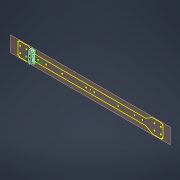
# Autodesk Inventor part: Home Switch Mount X
Saved by Autodesk Inventor 2022 (Build 260153000, 153)
## iProperties
Created: 2021-11-21
Part Number: Home Switch Mount X
Material: Generic
Document SubType Name: Modeling
Designer: nicol
Density: 1 g/cm^3
Appearance: Default
Author: nicol
Autodesk Inventor part; units mm, degrees
ref_plane "YZ Plane" through (0, 0, 0) normal (1, 0, 0) x (0, 1, 0)
ref_plane "XZ Plane" through (0, 0, 0) normal (0, 1, 0) x (-1, 0, 0)
ref_plane "XY Plane" through (0, 0, 0) normal (0, 0, 1) x (1, 0, 0)
ref_plane "Work Plane1" through (0, 0, 0) normal (0, 0, 1) x (1, 0, 0)
sketch "Sketch1" plane through (0, 0, 0) normal (0, 0, 1) x (1, 0, 0)
  line L0 (-193.5, -22) -> (-172.7154, -10) projected
  arc A0 (-226.5, -17.6844) -> (-226.2768, -18.2232) centre (-225.738, -17.6844) ccw projected
  line L1 (-222.7232, -21.7768) -> (-226.2768, -18.2232) projected
  arc A1 (-222.7232, -21.7768) -> (-222.1844, -22) centre (-222.1844, -21.238) ccw projected
  line L2 (-193.5, -22) -> (-222.1844, -22) projected
  line L3 (-193.5, -22) -> (-172.7154, -10) projected
  line L4 (-172.7154, -10) -> (172.7154, -10) projected
  line L5 (172.7154, -10) -> (193.5, -22) projected
  line L6 (193.5, -22) -> (222.1844, -22) projected
  arc A2 (222.1844, -22) -> (222.7232, -21.7768) centre (222.1844, -21.238) ccw projected
  line L7 (226.2768, -18.2232) -> (222.7232, -21.7768) projected
  arc A3 (226.2768, -18.2232) -> (226.5, -17.6844) centre (225.738, -17.6844) ccw projected
  line L8 (226.5, 17.6844) -> (226.5, -17.6844) projected
  arc A4 (226.5, 17.6844) -> (226.2768, 18.2232) centre (225.738, 17.6844) ccw projected
  line L9 (222.7232, 21.7768) -> (226.2768, 18.2232) projected
  arc A5 (222.7232, 21.7768) -> (222.1844, 22) centre (222.1844, 21.238) ccw projected
  line L10 (193.5, 22) -> (222.1844, 22) projected
  line L11 (193.5, 22) -> (172.7154, 10) projected
  line L12 (172.7154, 10) -> (-172.7154, 10) projected
  line L13 (-172.7154, 10) -> (-193.5, 22) projected
  line L14 (-193.5, 22) -> (-222.1844, 22) projected
  arc A6 (-222.1844, 22) -> (-222.7232, 21.7768) centre (-222.1844, 21.238) ccw projected
  line L15 (-226.2768, 18.2232) -> (-222.7232, 21.7768) projected
  arc A7 (-226.2768, 18.2232) -> (-226.5, 17.6844) centre (-225.738, 17.6844) ccw projected
  line L16 (-226.5, -17.6844) -> (-226.5, 17.6844) projected
  circle A8 centre (-13, 0) radius 1.2645 projected
  circle A9 centre (87, 0) radius 1.2645 projected
  circle A10 centre (-138, 0) radius 1.2645 projected
  circle A11 centre (162, 0) radius 1.2645 projected
  circle A12 centre (-163, 0) radius 1.2645 projected
  circle A13 centre (137, 0) radius 1.2645 projected
  circle A14 centre (-88, 0) radius 1.2645 projected
  circle A15 centre (12, 0) radius 1.2645 projected
  circle A16 centre (-200, -10) radius 1.7 projected
  circle A17 centre (-220, 10) radius 1.7 projected
  circle A18 centre (-220, -10) radius 1.7 projected
  circle A19 centre (-200, 10) radius 1.7 projected
  circle A20 centre (200, -10) radius 1.7 projected
  circle A21 centre (220, 10) radius 1.7 projected
  circle A22 centre (220, -10) radius 1.7 projected
  circle A23 centre (200, 10) radius 1.7 projected
  line L17 (-175, -5.5) -> (-175, 5.5) projected
  line L18 (-187.7, -18.6514) -> (-175, -18.6514)
  line L19 (-175, -18.6514) -> (-175, 18.6514)
  line L20 (-175, 18.6514) -> (-187.7, 18.6514)
  line L21 (-187.7, 18.6514) -> (-187.7, -18.6514)
  line L22 (-181.7, 18.6514) -> (-175, 14.7831)
  line L23 (-181.7, -18.6514) -> (-175, -14.7831)
  circle A24 centre (-181.7, -4.75) radius 1.35
  circle A25 centre (-181.7, 4.75) radius 1.35
  line L24 (-181.7, 4.75) -> (-181.7, -4.75) construction
  line L25 (-187.7, -18.6514) -> (-175, -11.319)
  line L26 (-175, 11.319) -> (-187.7, 18.6514)
  point P0 (0, 0)
  point P1 (-181.7, 0)
  point P2 (-175, 0)
  point P3 (-175, -11.319)
  dimension "d0" = 3
  dimension "d1" = 3
  dimension "d2" = 9.5
  dimension "d3" = 2.7
  dimension "d4" = 2.7
  dimension "d5" = 12.7
  constraints: 18 end point, 10 point on line, 4 parallel, 2 centre point, 2 collinear, 2 midpoint, 1 horizontal, 1 horizontal alignment, 1 perpendicular, 1 vertical, 1 vertical alignment
  measures "d0" distance between parallel lines of L13 L22
  measures "d1" distance between parallel lines of L23 L0
  measures "d2" distance of L24.end L24.start
  measures "d3" diameter of A25
  measures "d4" diameter of A24
  measures "d5" distance of L18.start L18.end
extrude "Extrusion1" add sketch "Sketch1" along normal blind 8 contours L21 L13 L19 L17 L0
extrude "Extrusion2" add sketch "Sketch1" along normal blind 8 and the other way blind 6 contours L0 L19 L23 L18 | L20 L22 L19 L13
chamfer "Chamfer1" distance 0.5 angle 45 2 edges at (-183.05, 4.75, 8) (-183.05, -4.75, 8)
equation "\"d1\" = d0"
equation "\"d4\" = d3"
body "Solid1"
